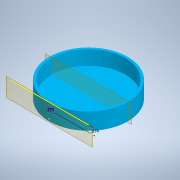
# Autodesk Inventor part: baseForBevelGearMount
Saved by Autodesk Inventor 2021 (Build 250183000, 183)
## iProperties
Created: 2020-06-18
Part Number: baseForBevelGearMount
Material: Polycarbonate, Clear
Document SubType Name: Modeling
Designer: robst
Density: 1.2 g/cm^3
Appearance: Sky Blue Medium
Author: robst
Autodesk Inventor part; units mm, degrees
ref_plane "YZ Plane" through (0, 0, 0) normal (1, 0, 0) x (0, 1, 0)
ref_plane "XZ Plane" through (0, 0, 0) normal (0, 1, 0) x (-1, 0, 0)
sketch "Sketch1" plane through (0, 0, 0) normal (0, 1, 0) x (-1, 0, 0)
  circle A0 centre (0, 0) radius 104.775
  dimension "d0" = 209.55
  constraints: 1 centre point, 1 coincident
  measures "d0" diameter of A0
extrude "Extrusion1" add sketch "Sketch1" against normal blind 6.35
sketch "Sketch2" plane through (0, 0, 0) normal (0, 1, 0) x (1, 0, 0)
  circle A0 centre (0, 0) radius 104.775 projected
  circle A1 centre (0, 0) radius 104.775
  circle A2 centre (0, 0) radius 98.425
  dimension "d3" = 6.35
  constraints: 2 centre point, 2 coincident, 1 concentric
  measures "d3" radial gap between concentric circles of A2 A0
extrude "Extrusion2" add sketch "Sketch2" along normal blind 38.1
ref_plane "Work Plane1" through (0, 0, 104.775) normal (0, 0, 1) x (1, 0, 0)
sketch "Sketch3" plane through (0, 0, 104.775) normal (0, 0, 1) x (1, 0, 0)
  circle A0 centre (0, 20.9804) radius 4.7625
  line L0 (104.775, 38.1) -> (-104.775, 38.1) projected
  point P0 (0, 0)
  dimension "d6" = 9.525
  dimension "d7" = 17.1196
  constraints: 1 centre point
  measures "d6" diameter of A0
  measures "d7" distance from line of A0.centre L0
extrude "Extrusion3" cut sketch "Sketch3" against normal through all
body "Solid1"
